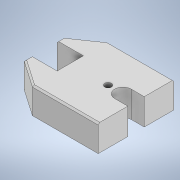
# Autodesk Inventor part: Ch7(5) Part 1 Base
Saved by Autodesk Inventor 2020 (Build 240168000, 168)
## iProperties
Created: 2021-02-25
Part Number: Ch7(5) Part 1 Base
Material: Generic
Document SubType Name: Modeling
Designer: adriggs
Density: 1 g/cm^3
Appearance: Default
Author: adriggs
Autodesk Inventor part; units mm, degrees
ref_plane "YZ Plane" through (0, 0, 0) normal (1, 0, 0) x (0, 1, 0)
ref_plane "XZ Plane" through (0, 0, 0) normal (0, 1, 0) x (-1, 0, 0)
ref_plane "XY Plane" through (0, 0, 0) normal (0, 0, 1) x (1, 0, 0)
sketch "Sketch1" plane through (0, 0, 0) normal (0, 1, 0) x (-1, 0, 0)
  line L0 (0, -51.1175) -> (0, 51.1175) projected
  line L1 (-17.78, 0) -> (106.68, 0) projected
  line L2 (106.68, 0) -> (-17.78, 0) projected
  line L3 (0, -51.1175) -> (0, 51.1175) projected
  line L4 (63.5, 36.5125) -> (0, 36.5125)
  line L5 (0, -36.5125) -> (63.5, -36.5125)
  line L6 (0, 36.5125) -> (63.5, 36.5125)
  line L7 (88.9, 18.9865) -> (63.5, 36.5125)
  line L8 (88.9, 12.6873) -> (63.5, 12.6873)
  line L9 (63.5, 12.6873) -> (63.5, 0)
  line L10 (88.9, -18.9865) -> (63.5, -36.5125)
  line L11 (88.9, -12.6873) -> (63.5, -12.6873)
  line L12 (63.5, -12.6873) -> (63.5, 0)
  line L13 (88.9, 18.9865) -> (88.9, 12.6873)
  line L14 (88.9, -12.6873) -> (88.9, -18.9865)
  line L15 (0, 7.9375) -> (12.6873, 7.9375)
  line L16 (12.6873, -7.9375) -> (0, -7.9375)
  arc A0 (12.6873, -7.9375) -> (12.6873, 7.9375) centre (12.6873, 0) ccw
  line L17 (0, 36.5125) -> (0, 7.9375)
  line L18 (0, -7.9375) -> (0, -36.5125)
  point P0 (0, 0)
  point P1 (0, 0)
  point P2 (0, 36.5125)
  point P3 (0, -7.9375)
  dimension "d1" = 73.025
  dimension "d2" = 63.5
  dimension "d4" = 17.526
  dimension "d5" = 88.9
  dimension "d7" = 23.8252
  dimension "d10" = 12.6873
  dimension "d11" = 15.875
  dimension "d12" = 36.5125
  constraints: 30 end point, 8 perpendicular, 6 vertical alignment, 5 symmetric about line, 4 point on line, 2 point on circle, 2 vertical, 1 centre point, 1 tangent, 6 other
  measures "d1" distance of L4.end L5.start
  measures "d2" distance of L4.start L4.end
  measures "d4" vertical distance of L4.start L7.start
  measures "d5" horizontal distance of L4.end L7.start
  measures "d7" vertical distance of L8.start L4.start
  measures "d10" horizontal distance of L15.start A0.centre
  measures "d11" distance of L16.end L15.start
  measures "d12" distance of point (0, 0) L4.end
extrude "Extrusion1" add sketch "Sketch1" along normal blind 25.4 contours L0 L16 A0 L1 L12 L11 L14 L10 L5 | L0 L4 L7 L13 L8 L9 L1 A0 L15
chamfer "Chamfer1" distance 1.524 angle 45 6 edges at (-31.75, 25.4, 36.5125) (-76.2, 25.4, 27.7495) (-88.9, 25.4, 15.8369) (-31.75, 25.4, -36.5125) (-76.2, 25.4, -27.7495) (-88.9, 25.4, -15.8369)
sketch "Sketch2" plane through (0, 25.4, 0) normal (0, 1, 0) x (1, 0, 0)
  point P0 (0, 0)
  point P1 (-26.9748, 0)
  dimension "d18" = 26.9748
  measures "d18" distance of point (0, 0) point (-26.975, 0)
hole "Hole1" at (-26.9748, 25.4, 0) direction (0, -1, 0) diameter 6.477 depth 14.2748 tip angle 118
sketch "Sketch3" plane through (-63.5, 0, -12.6873) normal (-1, 0, 0) x (0, 0, 1)
  line L0 (0, 0) -> (25.3746, 0) projected
  point P0 (12.6873, 0)
  point P1 (12.6873, 12.7)
  point P2 (12.6873, 0)
  dimension "d26" = 12.7
  constraints: 1 midpoint, 1 vertical alignment
  measures "d26" distance from line of point (12.687, 12.7) L0
hole "Hole2" at (-63.5, 12.7, 0) direction (1, 0, 0) diameter 7.7978 depth 19.05 tip angle 118 thread size "3/8-16 UNC" class "2B" standard "ANSI Unified Screw Threads"
body "Solid1"
